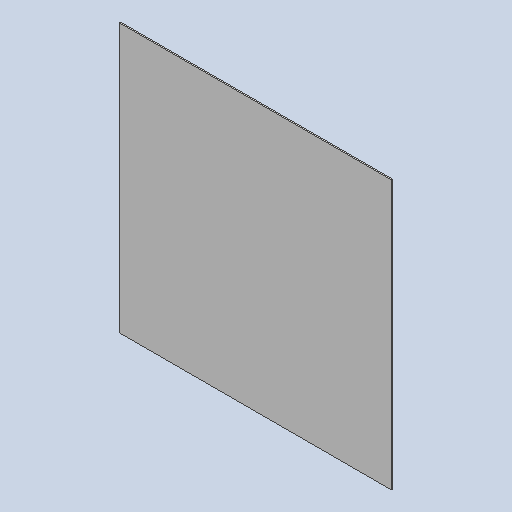
# Autodesk Inventor part: DF1.03 Wall bottom v2.0
Saved by Autodesk Inventor 2025 (Build 290162010, 162A)
## iProperties
Created: 2023-08-31
Part Number: DF1.03 Wall bottom v2.0
Material: Generic
Document SubType Name: Sheet Metal
Designer: admin
Density: 1 g/cm^3
Appearance: Default
Flat Pattern Width: 218 cm
Flat Pattern Length: 221 cm
Flat Pattern Area: 48178 cm^2
Sheet Metal Rule: Default
Sheet Metal Width: 2180,000 mm
Sheet Metal Length: 2210,000 mm
Sheet Metal Area: 4817800,000 mm^2
Author: admin
Autodesk Inventor part; units mm, degrees
ref_plane "YZ Plane" through (0, 0, 0) normal (1, 0, 0) x (0, 1, 0)
ref_plane "XZ Plane" through (0, 0, 0) normal (0, 1, 0) x (-1, 0, 0)
ref_plane "XY Plane" through (0, 0, 0) normal (0, 0, 1) x (1, 0, 0)
sketch "Sketch1" plane through (0, 0, 0) normal (0, 0, 1) x (1, 0, 0)
  line L0 (-1105, 1090) -> (1105, 1090)
  line L1 (1105, 1090) -> (1105, -1090)
  line L2 (1105, -1090) -> (-1105, -1090)
  line L3 (-1105, -1090) -> (-1105, 1090)
  line L4 (-1105, 1090) -> (1105, -1090) construction
  line L5 (1105, 1090) -> (-1105, -1090) construction
  point P0 (0, 0)
  dimension "d0" = 2180
  dimension "d1" = 2210
  constraints: 12 end point, 2 midpoint, 2 parallel, 1 horizontal, 1 perpendicular
  measures "d0" distance of L2.end L0.start
  measures "d1" distance of L1.end L2.end
extrude "Extrusion1" add sketch "Sketch1" along normal blind 10
equation "\"BendReliefDepth\" = 0.5 * Thickness"
equation "\"Thickness\" = 10"
body "Solid1"
